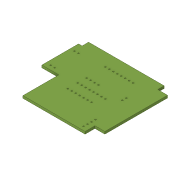
# Autodesk Inventor part: Main PCB2
Saved by Autodesk Inventor 2017 (Build 210142000, 142)
## iProperties
Created: 2016-12-21
Part Number: Main PCB2
Material: Generic
Document SubType Name: Modeling
Designer: ge937963
Density: 1 g/cm^3
Appearance: Olive Green
Author: ge937963
Autodesk Inventor part; units mm, degrees
ref_plane "YZ Plane" through (0, 0, 0) normal (1, 0, 0) x (0, 1, 0)
ref_plane "XZ Plane" through (0, 0, 0) normal (0, 1, 0) x (-1, 0, 0)
ref_plane "XY Plane" through (0, 0, 0) normal (0, 0, 1) x (1, 0, 0)
sketch "Sketch1" plane through (0, 0, 0) normal (0, 1, 0) x (-1, 0, 0)
  line L0 (38.3189, -53.1839) -> (-10.1951, -53.1839)
  line L1 (-10.1951, -53.1839) -> (-10.1951, -49.0183)
  line L2 (-10.1951, -49.0183) -> (-16.5451, -49.0183)
  line L3 (-16.5451, -49.0183) -> (-16.5451, -8.7339)
  line L4 (-16.5451, -8.7339) -> (-10.1951, -8.7339)
  line L5 (-10.1951, -8.7339) -> (-10.1951, -2.3839)
  line L6 (-10.1951, -2.3839) -> (29.6829, -2.3839)
  line L7 (29.6829, -2.3839) -> (29.6829, -25.4471)
  line L8 (29.6829, -25.4471) -> (40.6049, -25.4471)
  line L9 (40.6049, -25.4471) -> (40.6049, -49.0183)
  line L10 (40.6049, -49.0183) -> (38.3189, -49.0183)
  line L11 (38.3189, -49.0183) -> (38.3189, -53.1839)
  circle A0 centre (37.8363, -43.6589) radius 0.4445
  circle A1 centre (35.2963, -43.6589) radius 0.4445
  circle A2 centre (37.6077, -28.1395) radius 0.4445
  circle A3 centre (35.0677, -28.1395) radius 0.4445
  circle A4 centre (19.1165, -44.7765) radius 0.4445
  circle A5 centre (16.5765, -44.7765) radius 0.4445
  circle A6 centre (14.0365, -44.7765) radius 0.4445
  circle A7 centre (11.4965, -44.7765) radius 0.4445
  circle A8 centre (8.9565, -44.7765) radius 0.4445
  circle A9 centre (6.4165, -44.7765) radius 0.4445
  circle A10 centre (3.8765, -44.7765) radius 0.4445
  circle A11 centre (1.3365, -44.7765) radius 0.4445
  circle A12 centre (19.1165, -26.9965) radius 0.4445
  circle A13 centre (16.5765, -26.9965) radius 0.4445
  circle A14 centre (14.0365, -26.9965) radius 0.4445
  circle A15 centre (11.4965, -26.9965) radius 0.4445
  circle A16 centre (8.9565, -26.9965) radius 0.4445
  circle A17 centre (6.4165, -26.9965) radius 0.4445
  circle A18 centre (3.8765, -26.9965) radius 0.4445
  circle A19 centre (1.3365, -26.9965) radius 0.4445
  circle A20 centre (19.1165, -20.6465) radius 0.4445
  circle A21 centre (16.5765, -20.6465) radius 0.4445
  circle A22 centre (14.0365, -20.6465) radius 0.4445
  circle A23 centre (11.4965, -20.6465) radius 0.4445
  circle A24 centre (8.9565, -20.6465) radius 0.4445
  circle A25 centre (6.4165, -20.6465) radius 0.4445
  circle A26 centre (3.8765, -20.6465) radius 0.4445
  circle A27 centre (18.9387, -32.5591) radius 0.4445
  circle A28 centre (16.3987, -32.5591) radius 0.4445
  circle A29 centre (13.8587, -32.5591) radius 0.4445
  circle A30 centre (11.3187, -32.5591) radius 0.4445
  circle A31 centre (-6.9439, -4.6953) radius 0.4445
  circle A32 centre (-6.9439, -7.2353) radius 0.4445
  circle A33 centre (-6.9439, -9.7753) radius 0.4445
  circle A34 centre (-6.9439, -12.3153) radius 0.4445
  circle A35 centre (-4.9119, -31.5939) radius 0.4445
  circle A36 centre (-4.9119, -34.1339) radius 0.4445
  point P0 (0, 0)
  dimension "d0" = 57.15
  dimension "d1" = 50.8
  dimension "d2" = 4.1656
  dimension "d3" = 6.35
  dimension "d4" = 6.35
  dimension "d5" = 10.922
  dimension "d6" = 23.0632
  dimension "d7" = 2.286
  dimension "d8" = 0.889
  dimension "d9" = 2.54
  dimension "d10" = 2.7686
  dimension "d11" = 9.525
  dimension "d12" = 0.889
  dimension "d13" = 2.54
  dimension "d14" = 2.6924
  dimension "d15" = 2.9972
  dimension "d16" = 2.54
  dimension "d17" = 2.54
  dimension "d18" = 2.54
  dimension "d19" = 2.54
  dimension "d20" = 2.54
  dimension "d21" = 2.54
  dimension "d22" = 2.54
  dimension "d23" = 8.4074
  dimension "d24" = 21.4884
  dimension "d25" = 2.54
  dimension "d26" = 2.54
  dimension "d27" = 2.54
  dimension "d28" = 2.54
  dimension "d29" = 2.54
  dimension "d30" = 2.54
  dimension "d31" = 2.54
  dimension "d32" = 17.78
  dimension "d33" = 2.54
  dimension "d34" = 2.54
  dimension "d35" = 2.54
  dimension "d36" = 2.54
  dimension "d37" = 2.54
  dimension "d38" = 2.54
  dimension "d39" = 6.35
  dimension "d40" = 2.54
  dimension "d41" = 2.54
  dimension "d42" = 2.54
  dimension "d44" = 2.54
  dimension "d45" = 2.54
  dimension "d46" = 2.54
  dimension "d47" = 2.3114
  dimension "d48" = 3.2512
  dimension "d49" = 0.1778
  dimension "d50" = 5.5626
  dimension "d51" = 2.54
  dimension "d52" = 14.8844
  dimension "d53" = 11.6332
  constraints: 37 centre point, 32 equal radius, 27 horizontal alignment, 24 end point, 11 perpendicular, 6 vertical alignment, 1 horizontal
  measures "d0" distance between parallel lines of L3 L9
  measures "d1" distance between parallel lines of L6 L0
  measures "d2" distance of L0.end L1.end
  measures "d3" distance of L1.end L2.end
  measures "d4" distance of L4.end L5.end
  measures "d5" distance of L7.end L8.end
  measures "d6" distance of L6.end L7.end
  measures "d7" distance of L9.end L10.end
  measures "d8" diameter of A0
  measures "d9" distance of A1.centre A0.centre
  measures "d10" distance from line of L9 A0.centre
  measures "d11" vertical distance of L0.start A0.centre
  measures "d12" diameter of A2
  measures "d13" distance of A3.centre A2.centre
  measures "d14" vertical distance of L8.end A2.centre
  measures "d15" horizontal distance of L8.end A2.centre
  measures "d16" distance of A5.centre A4.centre
  measures "d17" distance of A6.centre A5.centre
  measures "d18" distance of A7.centre A6.centre
  measures "d19" distance of A8.centre A7.centre
  measures "d20" distance of A8.centre A9.centre
  measures "d21" distance of A9.centre A10.centre
  measures "d22" distance of A10.centre A11.centre
  measures "d23" distance from line of L0 A4.centre
  measures "d24" horizontal distance of L9.end A4.centre
  measures "d25" distance of A13.centre A12.centre
  measures "d26" distance of A14.centre A13.centre
  measures "d27" distance of A15.centre A14.centre
  measures "d28" distance of A16.centre A15.centre
  measures "d29" distance of A16.centre A17.centre
  measures "d30" distance of A17.centre A18.centre
  measures "d31" distance of A18.centre A19.centre
  measures "d32" distance of A12.centre A4.centre
  measures "d33" distance of A21.centre A20.centre
  measures "d34" distance of A22.centre A21.centre
  measures "d35" distance of A23.centre A22.centre
  measures "d36" distance of A24.centre A23.centre
  measures "d37" distance of A24.centre A25.centre
  measures "d38" distance of A25.centre A26.centre
  measures "d39" distance of A20.centre A12.centre
  measures "d40" distance of A28.centre A27.centre
  measures "d41" distance of A29.centre A28.centre
  measures "d42" distance of A30.centre A29.centre
  measures "d44" distance of A33.centre A34.centre
  measures "d45" distance of A33.centre A32.centre
  measures "d46" distance of A32.centre A31.centre
  measures "d47" vertical distance of L5.end A31.centre
  measures "d48" distance from line of A31.centre L5
  measures "d49" horizontal distance of A12.centre A27.centre
  measures "d50" vertical distance of A27.centre A12.centre
  measures "d51" distance of A35.centre A36.centre
  measures "d52" vertical distance of L2.end A36.centre
  measures "d53" horizontal distance of L2.end A36.centre
extrude "Extrusion1" add sketch "Sketch1" along normal blind 1.524
body "Solid1"
